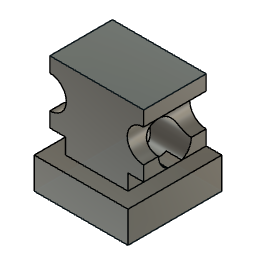
挂灯子 v1 (Autodesk Fusion 360 design; units mm, degrees)
Autodesk Fusion 360 part; units mm, degrees
sketch "草图1" plane through (0, 0, 0) normal (0, 0, 1) x (1, 0, 0)
  line L0 (0, 10) -> (6, 10)
  line L1 (6, 10) -> (6, 3.9983)
  line L2 (6, 3.9983) -> (0, 3.9983)
  line L3 (0, 3.9983) -> (0, 10)
  dimension "d1" = 6
  constraint horizontal L0
  constraint vertical L1
  constraint horizontal L2
  constraint vertical L3
  measures "d1" distance of L0.start L0.end
extrude "拉伸1" add sketch "草图1" along normal blind 2
sketch "草图2" plane through (0, 0, 0) normal (0, 0, -1) x (1, 0, 0)
  line L0 (6, -3.9983) -> (0, -3.9983)
  line L1 (0, -3.9983) -> (0, -10)
  line L2 (0, -10) -> (6, -10)
  line L3 (6, -10) -> (6, -3.9983)
sketch "草图3" plane through (0, 0, 0) normal (0, 0, -1) x (1, 0, 0)
  line L0 (5.5, -9.5) -> (0.5, -9.5)
  line L1 (0.5, -9.5) -> (0.5, -4.5)
  line L2 (0.5, -4.5) -> (5.5, -4.5)
  line L3 (5.5, -4.5) -> (5.5, -9.5)
  constraint horizontal L0
  constraint vertical L1
  constraint horizontal L2
  constraint vertical L3
extrude "拉伸2" cut sketch "草图3" against normal blind 1.5
sketch "草图4" plane through (0, 0, 2) normal (0, 0, 1) x (-1, 0, 0)
  line L0 (0, -3.9983) -> (-6, -3.9983)
  line L1 (-6, -3.9983) -> (-6, -10)
  line L2 (-6, -10) -> (0, -10)
  line L3 (0, -10) -> (0, -3.9983)
  line L4 (-5, -5) -> (-1, -5)
  line L5 (-1, -5) -> (-1, -9)
  line L6 (-1, -9) -> (-5, -9)
  line L7 (-5, -9) -> (-5, -5)
  constraint horizontal L4
  constraint vertical L5
  constraint horizontal L6
  constraint vertical L7
extrude "拉伸3" add sketch "草图4" along normal blind 1 contours L4 L5 L6 L7
sketch "草图5" plane through (0, 0, 3) normal (0, 0, 1) x (-1, 0, 0)
  line L0 (-5, -9) -> (-1, -9)
  line L1 (-1, -9) -> (-1, -5)
  line L2 (-1, -5) -> (-5, -5)
  line L3 (-5, -5) -> (-5, -9)
  line L4 (-6, -5) -> (0, -5)
  line L5 (0, -5) -> (0, -9)
  line L6 (0, -9) -> (-6, -9)
  line L7 (-6, -9) -> (-6, -5)
  constraint horizontal L4
  constraint vertical L5
  constraint horizontal L6
  constraint vertical L7
extrude "拉伸4" add sketch "草图5" along normal blind 4
hole "孔1" at (6, 9, 5) direction (0, -1, 0) diameter 2.1 depth 6.5 tip angle 118
hole "孔2" at (0, 9, 5) direction (0, -1, 0) diameter 2.1 depth 6.5 tip angle 118
hole "孔3" at (0, 7, 3.95) direction (1, 0, 0) diameter 2.1 depth 6.5 tip angle 118
sketch "草图6" plane through (0, 0, 7) normal (0, 0, 1) x (-1, 0, 0)
  line L0 (-6, -9) -> (0, -9)
  line L1 (0, -9) -> (0, -5)
  line L2 (0, -5) -> (-6, -5)
  line L3 (-6, -5) -> (-6, -9)
hole "孔4" at (2.9657, 7.0441, 1.5) direction (0, 0, 1) diameter 2 depth 4 tip angle 118
